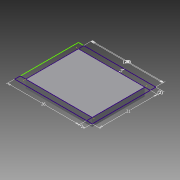
# Autodesk Inventor part: Pressure Regulator switch
Saved by Autodesk Inventor 2015 (Build 190159000, 159)
## iProperties
Created: 2019-01-09
Part Number: Pressure Regulator switch
Material: Generic
Document SubType Name: Modeling
Designer: 579494
Density: 1 g/cm^3
Appearance: Default
Author: 579494
Autodesk Inventor part; units mm, degrees
ref_plane "YZ Plane" through (0, 0, 0) normal (1, 0, 0) x (0, 1, 0)
ref_plane "XZ Plane" through (0, 0, 0) normal (0, 1, 0) x (-1, 0, 0)
ref_plane "XY Plane" through (0, 0, 0) normal (0, 0, 1) x (1, 0, 0)
sketch "Sketch1" plane through (0, 0, 0) normal (0, 0, 1) x (1, 0, 0)
  line L0 (0, 0) -> (24, 0)
  line L1 (24, 0) -> (24, 19)
  line L2 (24, 19) -> (0, 19)
  line L3 (0, 19) -> (0, 0)
  dimension "d0" = 24
  dimension "d1" = 19
  constraints: 8 end point, 2 parallel, 1 horizontal, 1 perpendicular
  measures "d0" distance of L2.end L1.end
  measures "d1" distance of L0.end L1.end
extrude "Extrusion1" add sketch "Sketch1" along normal blind 3
sketch "Sketch2" plane through (0, 0, 3) normal (0, 0, 1) x (1, 0, 0)
  line L0 (0, 19) -> (26, 19)
  line L1 (26, 19) -> (26, 21)
  line L2 (26, 21) -> (0, 21)
  line L3 (0, 21) -> (0, 19)
  line L4 (24, 19) -> (26, 19)
  line L5 (26, 19) -> (26, -2)
  line L6 (26, -2) -> (24, -2)
  line L7 (24, -2) -> (24, 19)
  line L8 (24, 0) -> (-2, 0)
  line L9 (-2, 0) -> (-2, -2)
  line L10 (-2, -2) -> (24, -2)
  line L11 (24, -2) -> (24, 0)
  line L12 (0, 19) -> (26, 19)
  line L13 (26, 19) -> (26, 21)
  line L14 (26, 21) -> (0, 21)
  line L15 (0, 21) -> (0, 19)
  line L16 (0, 19) -> (26, 19)
  line L17 (26, 19) -> (26, 21)
  line L18 (26, 21) -> (0, 21)
  line L19 (0, 21) -> (0, 19)
  line L20 (0, 19) -> (26, 19)
  line L21 (26, 19) -> (26, 21)
  line L22 (26, 21) -> (0, 21)
  line L23 (0, 21) -> (0, 19)
  line L24 (0, 0) -> (-2, 0)
  line L25 (-2, 0) -> (-2, 21)
  line L26 (-2, 21) -> (0, 21)
  line L27 (0, 21) -> (0, 0)
  dimension "d4" = 26
  dimension "d5" = 2
  dimension "d6" = 2
  dimension "d7" = 21
  dimension "d8" = 26
  dimension "d9" = 26
  dimension "d10" = 2
  dimension "d11" = 26
  dimension "d12" = 2
  dimension "d13" = 26
  dimension "d14" = 2
  constraints: 56 end point, 14 parallel, 7 horizontal, 7 perpendicular, 1 point on line
  measures "d4" distance of L2.end L1.end
  measures "d5" distance between parallel lines of L0 L2
  measures "d6" distance of L5.end L6.end
  measures "d7" distance of L4.end L5.end
  measures "d8" distance of L10.end L9.end
  measures "d9" distance of L14.end L1.end
  measures "d10" distance of L1.end L12.end
  measures "d11" distance of L18.end L1.end
  measures "d12" distance of L1.end L16.end
  measures "d13" distance of L22.end L1.end
  measures "d14" distance of L1.end L20.end
body "Solid1"
